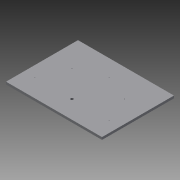
# Autodesk Inventor part: Shooter Base Plate
Saved by Autodesk Inventor 2013 (Build 170138000, 138)
## iProperties
Created: 2013-01-14
Part Number: Shooter Base Plate
Material: Generic
Document SubType Name: Modeling
Designer: carneeki
Density: 1 g/cm^3
Author: carneeki
Autodesk Inventor part; units mm, degrees
ref_plane "YZ Plane" through (0, 0, 0) normal (1, 0, 0) x (0, 1, 0)
ref_plane "XZ Plane" through (0, 0, 0) normal (0, 1, 0) x (-1, 0, 0)
ref_plane "XY Plane" through (0, 0, 0) normal (0, 0, 1) x (1, 0, 0)
sketch "Sketch1" plane through (0, 0, 0) normal (0, 1, 0) x (-1, 0, 0)
  line L0 (508, -571.5) -> (-508, -571.5)
  line L1 (-508, -571.5) -> (-508, 190.5)
  line L2 (-508, 190.5) -> (508, 190.5)
  line L3 (508, 190.5) -> (508, -571.5)
  circle A0 centre (0, 0) radius 14.2875
  line L4 (508, 0) -> (-508, 0) construction
  arc A1 (-393.7, 0) -> (393.7, 0) centre (0, 0) ccw construction
  circle A2 centre (393.7, 0) radius 3.175
  circle A3 centre (0, -393.7) radius 3.175
  circle A4 centre (-393.7, 0) radius 3.175
  circle A5 centre (278.3879, -278.3879) radius 3.175
  line L5 (0, 0) -> (278.3879, -278.3879) construction
  circle A6 centre (-278.3879, -278.3879) radius 3.175
  line L6 (-278.3879, -278.3879) -> (0, 0) construction
  dimension "d0" = 1016
  dimension "d2" = 762
  dimension "d4" = 508
  dimension "d5" = 28.575
  dimension "d9" = 787.4
  dimension "d10" = 393.7
  dimension "d11" = 508
  dimension "d12" = 6.35
  dimension "d13" = 6.35
  dimension "d14" = 6.35
  dimension "d15" = 6.35
  dimension "d16" = 45
  dimension "d17" = 6.35
  dimension "d18" = 45
  dimension "d19" = 571.5
  constraints: 14 end point, 7 centre point, 2 parallel, 2 point on circle, 2 point on line, 1 coincident, 1 horizontal, 1 perpendicular
  measures "d0" distance of L0.start L0.end
  measures "d2" distance of L2.end L0.start
  measures "d4" distance from line of point (0, 0) L3
  measures "d5" diameter of A0
  measures "d9" distance of A1.end A1.start
  measures "d10" radius of A1
  measures "d11" distance from line of L3 A1.centre
  measures "d12" diameter of A2
  measures "d13" diameter of A3
  measures "d14" diameter of A4
  measures "d15" diameter of A5
  measures "d16" angle of L5 L4
  measures "d17" diameter of A6
  measures "d18" angle of L4 L6
  measures "d19" distance from line of point (0, 0) L0
extrude "Extrusion1" add sketch "Sketch1" against normal blind 25.4
equation "\"d4\" = 0.5 * d0"
equation "\"d19\" = 0.75 * d2"
body "Solid1"
